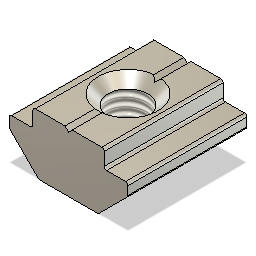
Slider T-Nut for 2020 - M4 (Autodesk Fusion 360 design; units mm, degrees)
Autodesk Fusion 360 part; units mm, degrees
sketch "Sketch1" plane through (0, 0, 0) normal (0, 0, 1) x (1, 0, 0)
  line L0 (2.6252, 0) -> (7.4595, 0)
  line L1 (10.0424, 2.5828) -> (10.0424, 3.3)
  line L2 (0.0424, 3.3) -> (0.0424, 2.5828)
  line L3 (8.0424, 3.7) -> (8.0424, 4.8)
  line L4 (2.0424, 4.8) -> (2.0424, 3.7)
  line L5 (0.101, 2.4414) -> (2.4838, 0.0586)
  line L6 (0.0424, 2.5) -> (3.5052, 2.5) construction
  line L7 (5.0424, 3.5) -> (5.0424, 0) construction
  line L8 (9.9838, 2.4414) -> (7.601, 0.0586)
  line L9 (9.8424, 3.5) -> (8.2424, 3.5)
  line L10 (1.8424, 3.5) -> (0.2424, 3.5)
  line L11 (5.0424, 4.7) -> (5.3424, 5)
  line L12 (5.0424, 4.7) -> (6.213, 4.7) construction
  line L13 (5.0424, 4.7) -> (4.7424, 5)
  line L14 (5.0424, 4.7) -> (6.2088, 4.7) construction
  line L15 (7.8424, 5) -> (5.3424, 5)
  line L16 (4.7424, 5) -> (2.2424, 5)
  arc A0 (0.2424, 3.5) -> (0.0424, 3.3) centre (0.2424, 3.3) ccw
  arc A1 (0.0424, 2.5828) -> (0.101, 2.4414) centre (0.2424, 2.5828) ccw
  arc A2 (2.4838, 0.0586) -> (2.6252, 0) centre (2.6252, 0.2) ccw
  arc A3 (7.4595, 0) -> (7.601, 0.0586) centre (7.4595, 0.2) ccw
  arc A4 (9.9838, 2.4414) -> (10.0424, 2.5828) centre (9.8424, 2.5828) ccw
  arc A5 (10.0424, 3.3) -> (9.8424, 3.5) centre (9.8424, 3.3) ccw
  arc A6 (8.0424, 3.7) -> (8.2424, 3.5) centre (8.2424, 3.7) ccw
  arc A7 (8.0424, 4.8) -> (7.8424, 5) centre (7.8424, 4.8) ccw
  arc A8 (2.2424, 5) -> (2.0424, 4.8) centre (2.2424, 4.8) ccw
  arc A9 (1.8424, 3.5) -> (2.0424, 3.7) centre (1.8424, 3.7) ccw
  dimension "d1" = 10
  dimension "d4" = 5
  dimension "d5" = 45
  dimension "d6" = 1
  dimension "d7" = 5
  dimension "d8" = 6
  dimension "d9" = 2
  dimension "d10" = 2
  dimension "d12" = 45
  dimension "d13" = 0.3
  dimension "d14" = 5
  dimension "d15" = 1.5
  dimension "d16" = 0.2
  measures "d1" distance of L1 L2
  measures "d4" distance of L0 L15
  measures "d5" angle of L5 L6
  measures "d6" distance of L9
  measures "d8" distance of L3 L4
  measures "d12" angle of L11 L12
  measures "d14" distance of L0 L16
  measures "d15" distance of L10 L16
  measures "d16" radius of A0
extrude "Extrude1" add sketch "Sketch1" along normal blind 10
hole "Hole1" at (5.0424, 5, 5) direction (0, -1, 0) diameter 3.332 depth 5.5 tip angle 180 countersink diameter 5 countersink angle 90
thread "Thread1" "ISO Metric profile 4.0 M4x0.7 6H"
